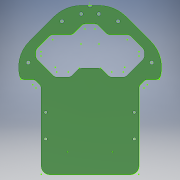
# Autodesk Inventor part: mainpcb
Saved by Autodesk Inventor 2018 (Build 220112000, 112)
## iProperties
Created: 2017-05-27
Part Number: mainpcb
Material: Ogólny
Document SubType Name: Modeling
Designer: Karol
Density: 1 g/cm^3
Appearance: Smooth - Dark Forest Green
Author: Karol
Autodesk Inventor part; units mm, degrees
ref_plane "YZ Plane" through (0, 0, 0) normal (1, 0, 0) x (0, 1, 0)
ref_plane "XZ Plane" through (0, 0, 0) normal (0, 1, 0) x (-1, 0, 0)
ref_plane "XY Plane" through (0, 0, 0) normal (0, 0, 1) x (1, 0, 0)
sketch "Sketch1" plane through (0, 0, 0) normal (0, 1, 0) x (-1, 0, 0)
  line L0 (0, 0) -> (0, -22.5)
  line L1 (5, -27.5) -> (48.7574, -27.5)
  arc A0 (0, -22.5) -> (5, -27.5) centre (5, -22.5) ccw
  arc A1 (89.1353, -20) -> (95.1955, -5) centre (73.6017, -5) ccw
  line L2 (89.1353, -20) -> (74.9931, -34.1421)
  line L3 (95.1955, -5) -> (95.1955, 0)
  line L4 (50.8787, -28.3787) -> (52.6569, -30.1569)
  line L5 (53.5355, -32.2782) -> (53.5355, -36.7771)
  arc A2 (55.8844, -39.7056) -> (74.9931, -34.1421) centre (60.372, -19.521) ccw
  line L6 (55.7045, -20.8787) -> (64.6301, -29.805)
  line L7 (66.7515, -30.6838) -> (69.1812, -30.6838)
  arc A3 (69.1812, -30.6838) -> (71.3027, -29.805) centre (69.1812, -27.6838) ccw
  arc A4 (64.6301, -29.805) -> (66.7515, -30.6838) centre (66.7515, -27.6838) ccw
  arc A5 (54.8259, -18.7574) -> (55.7045, -20.8787) centre (57.8259, -18.7574) ccw
  arc A6 (50.8787, -28.3787) -> (48.7574, -27.5) centre (48.7574, -30.5) ccw
  arc A7 (53.5355, -32.2782) -> (52.6569, -30.1569) centre (50.5355, -32.2782) ccw
  arc A8 (53.5355, -36.7771) -> (55.8844, -39.7056) centre (56.5355, -36.7771) ccw
  line L8 (71.3027, -29.805) -> (78.0002, -23.1064)
  line L9 (78.8787, -20.9852) -> (78.8787, -11.3601)
  line L10 (79.7568, -9.2393) -> (84.1169, -4.8769)
  arc A9 (78.0002, -23.1064) -> (78.8787, -20.9852) centre (75.8787, -20.9852) ccw
  arc A10 (79.7568, -9.2393) -> (78.8787, -11.3601) centre (81.8787, -11.3601) ccw
  arc A11 (84.1169, -4.8769) -> (84.995, -2.7562) centre (81.995, -2.7562) ccw
  line L11 (84.995, -2.7562) -> (84.995, 0)
  line L12 (59.826, 0) -> (59.826, -4.7574)
  line L13 (58.9473, -6.8787) -> (55.7046, -10.1214)
  line L14 (54.8259, -18.7574) -> (54.8259, -12.2428)
  arc A12 (55.7046, -10.1214) -> (54.8259, -12.2428) centre (57.8259, -12.2428) ccw
  arc A13 (58.9473, -6.8787) -> (59.826, -4.7574) centre (56.826, -4.7574) ccw
  line L15 (27.5, -24.9983) -> (27.5, -6.8787)
  line L16 (12.7, -25) -> (12.7, -12.5)
  line L17 (42.3, -12.5) -> (42.3, -25)
  line L18 (0, 0) -> (0, 22.5)
  arc A14 (5, 27.5) -> (0, 22.5) centre (5, 22.5) ccw
  arc A15 (52.6569, 30.1569) -> (53.5355, 32.2782) centre (50.5355, 32.2782) ccw
  line L19 (53.5355, 32.2782) -> (53.5355, 36.7771)
  arc A16 (55.8844, 39.7056) -> (53.5355, 36.7771) centre (56.5355, 36.7771) ccw
  arc A17 (66.7515, 30.6838) -> (64.6301, 29.805) centre (66.7515, 27.6838) ccw
  arc A18 (74.9931, 34.1421) -> (55.8844, 39.7056) centre (60.372, 19.521) ccw
  arc A19 (78.8787, 20.9852) -> (78.0002, 23.1064) centre (75.8787, 20.9852) ccw
  line L20 (89.1353, 20) -> (74.9931, 34.1421)
  line L21 (71.3027, 29.805) -> (78.0002, 23.1064)
  arc A20 (71.3027, 29.805) -> (69.1812, 30.6838) centre (69.1812, 27.6838) ccw
  line L22 (66.7515, 30.6838) -> (69.1812, 30.6838)
  line L23 (50.8787, 28.3787) -> (52.6569, 30.1569)
  line L24 (55.7045, 20.8787) -> (64.6301, 29.805)
  arc A21 (55.7045, 20.8787) -> (54.8259, 18.7574) centre (57.8259, 18.7574) ccw
  arc A22 (48.7574, 27.5) -> (50.8787, 28.3787) centre (48.7574, 30.5) ccw
  line L25 (78.8787, 20.9852) -> (78.8787, 11.3601)
  arc A23 (78.8787, 11.3601) -> (79.7568, 9.2393) centre (81.8787, 11.3601) ccw
  line L26 (79.7568, 9.2393) -> (84.1169, 4.8769)
  arc A24 (84.995, 2.7562) -> (84.1169, 4.8769) centre (81.995, 2.7562) ccw
  line L27 (84.995, 2.7562) -> (84.995, 0)
  line L28 (27.5, 24.9983) -> (27.5, 6.8787)
  line L29 (5, 27.5) -> (48.7574, 27.5)
  line L30 (54.8259, 18.7574) -> (54.8259, 12.2428)
  arc A25 (54.8259, 12.2428) -> (55.7046, 10.1214) centre (57.8259, 12.2428) ccw
  line L31 (58.9473, 6.8787) -> (55.7046, 10.1214)
  line L32 (59.826, 0) -> (59.826, 4.7574)
  arc A26 (59.826, 4.7574) -> (58.9473, 6.8787) centre (56.826, 4.7574) ccw
  arc A27 (95.1955, 5) -> (89.1353, 20) centre (73.6017, 5) ccw
  line L33 (95.1955, 5) -> (95.1955, 0)
  line L34 (12.7, 25) -> (12.7, 12.5)
  line L35 (42.3, 12.5) -> (42.3, 25)
  line L36 (59.826, 0) -> (0, 0)
  point P0 (0, -27.5)
  point P1 (35, -24.9983)
  point P2 (73.6017, -5)
  point P3 (53.5355, -31.0355)
  point P4 (53.5355, -39.0355)
  point P5 (70.4238, -30.6838)
  point P6 (54.8259, -20)
  point P7 (65.5088, -30.6838)
  point P8 (73.6017, -5)
  point P9 (73.6017, -5)
  point P10 (73.6017, -5)
  point P11 (73.6017, -5)
  point P12 (73.6017, -5)
  point P13 (73.6017, -5)
  point P14 (84.995, -3.9983)
  point P15 (59.826, -6)
  point P16 (63.036, -34.776)
  point P17 (86.3487, -15.8276)
  point P18 (90.4692, -5.0078)
  point P19 (20, -24.9983)
  point P20 (0, 27.5)
  point P21 (65.5088, 30.6838)
  point P22 (53.5355, 39.0355)
  point P23 (70.4238, 30.6838)
  point P24 (53.5355, 31.0355)
  point P25 (54.8259, 20)
  point P26 (73.6017, 5)
  point P27 (73.6017, 5)
  point P28 (73.6017, 5)
  point P29 (73.6017, 5)
  point P30 (73.6017, 5)
  point P31 (73.6017, 5)
  point P32 (73.6017, 5)
  point P33 (84.995, 3.9983)
  point P34 (59.826, 6)
  point P35 (20, 24.9983)
  point P36 (90.4692, 5.0078)
  point P37 (86.3487, 15.8276)
  point P38 (63.036, 34.776)
  point P39 (35, 24.9983)
  constraints: 74 end point, 58 point on circle, 28 centre point, 24 point on line, 2 vertical, 1 horizontal
extrude "Wyciągnięcie proste3" add sketch "Sketch1" along normal blind 1.4
hole "Otwór6" at (-95.1955, 0, 0) at (-90.4692, 0, -5.0078) at (-86.3487, 0, -15.8276) at (-63.036, 0, -34.776) at (-63.036, 0, 34.776) at (-86.3487, 0, 15.8276) at (-90.4692, 0, 5.0078) direction (0, 1, 0) diameter 2.5 end through all
hole "Otwór7" at (-20, 0, -24.9983) at (-35, 0, 24.9983) at (-20, 0, 24.9983) at (-35, 0, -24.9983) direction (0, 1, 0) diameter 2 end through all
hole "Otwór8" at (-12.7, 0, -12.5) at (-12.7, 0, 12.5) direction (0, 1, 0) diameter 1 end through all
